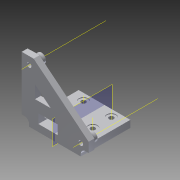
# Autodesk Inventor part: camera_support_prz
Saved by Autodesk Inventor 2015 SP1 (Build 190203100, 203)
## iProperties
Created: 2015-08-07
Part Number: camera_support_prz
Material: ABS Plastic
Document SubType Name: Modeling
Designer: Alexandre Cherpillod
Mass: 21 g
Surface Area: 23.8987 cm^2
Volume: 2.4271 cm^3
Density: 8.65231 g/cm^3
Appearance: Smooth - White
Author: Alexandre Cherpillod
Autodesk Inventor part; units mm, degrees
ref_plane "YZ Plane" through (0, 0, 0) normal (1, 0, 0) x (0, 1, 0)
ref_plane "XZ Plane" through (0, 0, 0) normal (0, 1, 0) x (-1, 0, 0)
ref_plane "XY Plane" through (0, 0, 0) normal (0, 0, 1) x (1, 0, 0)
sketch "Sketch1" plane through (0, 0, 0) normal (0, 1, 0) x (-1, 0, 0)
  line L0 (0, 0) -> (26.25, 0) construction
  line L1 (26.25, 0) -> (26.25, -22) construction
  line L2 (26.25, -22) -> (0, -22) construction
  line L3 (0, -22) -> (0, 0) construction
  circle A0 centre (2, -20) radius 1.95
  circle A1 centre (24.25, -2) radius 2
  dimension "d0" = 26.25
  dimension "d1" = 22
  dimension "d3" = 3.9
  dimension "d6" = 4
  dimension "d18" = 2
  dimension "d19" = 2
  dimension "d20" = 2
  dimension "d21" = 2
  constraints: 8 end point, 2 centre point, 2 parallel, 1 horizontal, 1 perpendicular
  measures "d0" distance of L1.end L2.end
  measures "d1" distance of L0.end L1.end
  measures "d3" diameter of A0
  measures "d6" diameter of A1
  measures "d18" distance from line of L1 A1.centre
  measures "d19" distance from line of L0 A1.centre
  measures "d20" distance from line of L3 A0.centre
  measures "d21" distance from line of L2 A0.centre
extrude "Extrusion1" add sketch "Sketch1" along normal blind 2.8
sketch "Sketch6" plane through (-24.25, 0, -2) normal (0, -1, 0) x (1, 0, 0)
  circle A0 centre (0, 0) radius 2 construction
  circle A1 centre (22.25, -18) radius 1.95 construction
  line L0 (-7.7702, -20) -> (30.063, -20) construction
  line L1 (1.9389, 3.3329) -> (25.6312, -15.8338)
  line L2 (25.6312, -15.8338) -> (25.6312, -20)
  circle A2 centre (22.25, -18) radius 1.95 projected
  line L3 (4, -20) -> (4, -16)
  line L4 (4, -16) -> (12.25, -16)
  line L5 (12.25, -16) -> (12.25, -20)
  line L6 (25.6312, -20) -> (12.25, -20)
  line L7 (4, -20) -> (-3.1908, -20)
  line L8 (2.5513, -5.9922) -> (9.3088, -11.459)
  line L9 (9.3088, -11.459) -> (2.5513, -11.459)
  line L10 (2.5513, -11.459) -> (2.5513, -5.9922)
  line L11 (-3.1908, -20) -> (-3.1908, 3.3329)
  line L12 (1.9389, 3.3329) -> (-3.1908, 3.3329)
  point P0 (24.25, 2)
  dimension "d28" = 2
  dimension "d31" = 10
  dimension "d32" = 4
  dimension "d40" = 4
  constraints: 26 end point, 5 perpendicular, 2 horizontal, 2 point on line, 2 vertical
  measures "d28" distance from line of L0 A1.centre
  measures "d31" distance from line of A1.centre L5
  measures "d32" distance between parallel lines of L0 L4
  measures "d40" distance from line of L3 A0.centre
extrude "Extrusion6" add sketch "Sketch6" along normal blind 2.5 contours L1 L2 L6 L5 L4 L3 L7 L11 L12 | A2
fillet "Fillet1" radius 2 1 edges at (-22.25, 0, -2)
hole "Hole1" at (-24.25, 2.8, -2) direction (0, -1, 0) diameter 2 depth 8 tip angle 118
hole "Hole2" at (-2, 2.8, -20) direction (0, -1, 0) diameter 2 depth 8 tip angle 118
fillet "Fillet2" radius 2 1 edges at (-0.05, 0, -20)
sketch "Sketch10" plane through (1.3812, -2.5, -22) normal (0, 0, -1) x (-1, 0, 0)
  line L0 (25.6312, -4.2658) -> (25.6312, 25.595) construction
  line L1 (3.3812, -4.2658) -> (3.3812, 25.595) construction
  line L2 (0, 0) -> (23.6922, 0) projected
  line L3 (3.3812, 0) -> (25.6312, 0)
  line L4 (25.6312, 0) -> (25.6312, 21.3292)
  line L5 (25.6312, 21.3292) -> (3.3812, 21.3292)
  line L6 (3.3812, 21.3292) -> (3.3812, 0)
  point P0 (1.3812, 2.5)
  constraints: 8 end point, 3 point on line, 2 parallel, 1 horizontal, 1 perpendicular
extrude "Extrusion8" add sketch "Sketch10" along normal blind 3
fillet "Fillet3" radius 2 1 edges at (-2, -0.4722, -22)
fillet "Fillet4" radius 2 1 edges at (-24.25, -1.25, -22)
fillet "Fillet5" radius 2 1 edges at (-22.25, 0, -22)
sketch "Sketch12" plane through (1.3812, -2.5, -22) normal (0, 0, 1) x (1, 0, 0)
  line L0 (-23.6312, 5.3) -> (-27.6312, 5.3) construction
  line L1 (-1.4312, 5.3) -> (-5.3312, 5.3) construction
  circle A0 centre (-20.5062, 18.3) radius 2
  circle A1 centre (-20.5062, 10.3) radius 2
  line L2 (-25.6312, 4.5) -> (-25.6312, 21.3292) projected
  line L3 (-3.3812, 21.3292) -> (-3.3812, 0) construction
  line L4 (-3.3812, 12.9146) -> (-25.6312, 12.9146) construction
  line L5 (-14.5062, 12.9146) -> (-14.5062, 6.5641) construction
  circle A2 centre (-8.5062, 18.3) radius 2
  circle A3 centre (-8.5062, 10.3) radius 2
  point P0 (-1.3812, 2.5)
  dimension "d67" = 4
  dimension "d70" = 5.125
  dimension "d72" = 5
  dimension "d73" = 5.125
  dimension "d112" = 12
  dimension "d113" = 8
  constraints: 4 centre point, 4 end point, 2 coincident, 2 midpoint, 2 symmetric about line, 1 point on line, 1 vertical, 2 other
  measures "d67" diameter of A0
  measures "d70" distance from line of A0.centre L2
  measures "d72" distance from line of L0 A1.centre
  measures "d73" distance from line of L2 A1.centre
  measures "d112" distance of A1.centre A3.centre
  measures "d113" distance of A0.centre A1.centre
extrude "Extrusion9" cut sketch "Sketch12" against normal blind 0.3
hole "Hole3" at (-19.125, 7.8, -22.3) direction (0, 0, -1) diameter 2 depth 8 tip angle 118
hole "Hole4" at (-19.125, 15.8, -22.3) direction (0, 0, -1) diameter 2 depth 8 tip angle 118
hole "Hole5" at (-7.125, 15.8, -22.3) direction (0, 0, -1) diameter 2 depth 8 tip angle 118
hole "Hole6" at (-7.125, 7.8, -22.3) direction (0, 0, -1) diameter 2 depth 8 tip angle 118
ref_plane "Work Plane3" through (-13.125, 7.8, -26.3) normal (-1, 0, 0) x (0, 0, 1)
ref_plane "Work Plane1" through (-7.125, 15.8, -26.3) normal (1, 0, 0) x (0, 0, 1)
ref_plane "Work Plane2" through (-19.125, 7.8, -26.3) normal (-1, 0, 0) x (0, 0, 1)
body "Solid1"
